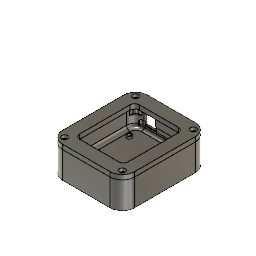
box (Autodesk Fusion 360 design; units mm, degrees)
Autodesk Fusion 360 part; units mm, degrees
sketch "Sketch1" plane through (0, 0, 2.8) normal (0, 0, 1) x (-1, 0, 0)
  circle A0 centre (-2.5, -2.5) radius 1.15 construction
  circle A1 centre (-48.5, -2.5) radius 1.15 construction
  circle A2 centre (-48.5, -61.5) radius 1.15 construction
  circle A3 centre (-2.5, -61.5) radius 1.15 construction
  line L0 (-2.5, -73.5) -> (-48.5, -73.5)
  line L1 (-60.5, -61.5) -> (-60.5, -2.5)
  line L2 (-48.5, 9.5) -> (-2.5, 9.5)
  line L3 (9.5, -2.5) -> (9.5, -61.5)
  arc A4 (-2.5, -73.5) -> (9.5, -61.5) centre (-2.5, -61.5) ccw
  arc A5 (-60.5, -61.5) -> (-48.5, -73.5) centre (-48.5, -61.5) ccw
  arc A6 (-48.5, 9.5) -> (-60.5, -2.5) centre (-48.5, -2.5) ccw
  arc A7 (9.5, -2.5) -> (-2.5, 9.5) centre (-2.5, -2.5) ccw
  arc A8 (-2.5, -7.5) -> (-6.5, -3.5) centre (-6.5, -7.5) ccw
  line L4 (-6.5, -3.5) -> (-44.5, -3.5)
  arc A9 (-44.5, -3.5) -> (-48.5, -7.5) centre (-44.5, -7.5) ccw
  line L5 (-48.5, -7.5) -> (-48.5, -56.5)
  arc A10 (-48.5, -56.5) -> (-44.5, -60.5) centre (-44.5, -56.5) ccw
  line L6 (-44.5, -60.5) -> (-6.5, -60.5)
  arc A11 (-6.5, -60.5) -> (-2.5, -56.5) centre (-6.5, -56.5) ccw
  line L7 (-2.5, -56.5) -> (-2.5, -7.5)
  line L8 (-44.5, -61) -> (-6.5, -61)
  arc A12 (-6.5, -61) -> (-2, -56.5) centre (-6.5, -56.5) ccw
  line L9 (-2, -56.5) -> (-2, -7.5)
  arc A13 (-2, -7.5) -> (-6.5, -3) centre (-6.5, -7.5) ccw
  line L10 (-6.5, -3) -> (-44.5, -3)
  arc A14 (-44.5, -3) -> (-49, -7.5) centre (-44.5, -7.5) ccw
  line L11 (-49, -7.5) -> (-49, -56.5)
  arc A15 (-49, -56.5) -> (-44.5, -61) centre (-44.5, -56.5) ccw
  circle A16 centre (-2.5, -61.5) radius 1.25
  circle A17 centre (-48.5, -61.5) radius 1.25
  circle A18 centre (-48.5, -2.5) radius 1.25
  circle A19 centre (-2.5, -2.5) radius 1.25
  dimension "d1" = 12
  dimension "d3" = 0.5
  dimension "d6" = 2.5
  dimension "d7" = 2.5
  dimension "d8" = 2.5
  dimension "d9" = 2.5
  measures "d1" radius of A4
  measures "d6" diameter of A16
  measures "d7" diameter of A17
  measures "d8" diameter of A19
  measures "d9" diameter of A18
extrude "Extrude1" add sketch "Sketch1" along normal blind 4.5 contours L0 L1 L2 L3 A4 A5 A6 A7 | A16 | A17 | A18 | A19 makes body 1
extrude "Extrude2" cut sketch "Sketch1" along normal blind 3.4 contours A16 | A17 | A18 | A19 bodies 1
ref_plane "WorkPlane1" through (25.5, 32, -23.2) normal (0, 0, -1) x (1, 0, 0)
sketch "Sketch2" plane through (25.5, 32, -23.2) normal (0, 0, -1) x (1, 0, 0)
  arc A0 (-35, -29.5) -> (-23, -41.5) centre (-23, -29.5) ccw
  line L0 (-23, -41.5) -> (23, -41.5)
  arc A1 (23, -41.5) -> (35, -29.5) centre (23, -29.5) ccw
  line L1 (35, -29.5) -> (35, 29.5)
  arc A2 (35, 29.5) -> (23, 41.5) centre (23, 29.5) ccw
  line L2 (23, 41.5) -> (-23, 41.5)
  arc A3 (-23, 41.5) -> (-35, 29.5) centre (-23, 29.5) ccw
  line L3 (-35, 29.5) -> (-35, -29.5)
extrude "Extrude3" add sketch "Sketch2" against normal up to surface (26 mm away) separate body makes body 2
shell "Shell1" thickness 3 removed faces 1 at (37.1667, 22.1667, 2.8) on bodies 2
fillet "Fillet1" radius 3.5 8 edges at (-3.864, -3.864, -20.2) (-6.5, 32, -20.2) (-3.864, 67.864, -20.2) (25.5, 70.5, -20.2) (54.864, 67.864, -20.2) (57.5, 32, -20.2) (54.864, -3.864, -20.2) (25.5, -6.5, -20.2) on bodies 2
ref_plane "WorkPlane2" through (25.5, 32, -18.2) normal (0, 0, 1) x (-1, 0, 0)
ref_plane "WorkPlane3" through (25.5, 32, -10.2) normal (1, 0, 0) x (0, 1, 0)
sketch "Sketch3" plane through (25.5, 32, -18.2) normal (0, 0, 1) x (1, 0, 0)
  line L0 (26.65, -26.3) -> (26.65, 38)
  arc A0 (26.65, 38) -> (26.15, 38.5) centre (26.15, 38) ccw
  line L1 (26.15, 38.5) -> (13.95, 38.5)
  line L2 (9.35, 38.5) -> (-13.85, 38.5)
  line L3 (-22.85, 38.5) -> (-26.15, 38.5)
  line L4 (-26.65, 38) -> (-26.65, -27)
  arc A1 (-26.15, 38.5) -> (-26.65, 38) centre (-26.15, 38) ccw
  line L5 (-22.85, 38.5) -> (-13.85, 38.5)
  line L6 (9.35, 38.5) -> (13.95, 38.5)
  line L7 (27.85, -26.3) -> (27.85, 38)
  arc A2 (27.85, 38) -> (26.15, 39.7) centre (26.15, 38) ccw
  line L8 (26.15, 39.7) -> (13.95, 39.7)
  line L9 (9.35, 39.7) -> (13.95, 39.7)
  line L10 (9.35, 39.7) -> (-13.85, 39.7)
  line L11 (-22.85, 39.7) -> (-13.85, 39.7)
  line L12 (-22.85, 39.7) -> (-26.15, 39.7)
  arc A3 (-26.15, 39.7) -> (-27.85, 38) centre (-26.15, 38) ccw
  line L13 (-27.85, 38) -> (-27.85, -27)
  line L14 (26.65, -26.3) -> (27.85, -26.3)
  line L15 (-27.85, -27) -> (-26.65, -27)
  line L16 (26.65, -26.3) -> (-26.65, -27)
  dimension "d26" = 1.2
extrude "Extrude4" cut sketch "Sketch3" along normal blind 5 bodies 2
sketch "Sketch4" plane through (0, 73.5, 0) normal (0, 1, 0) x (-1, 0, 0)
  line L0 (-2.65, -16.4) -> (-2.65, -4.9) construction
  line L1 (-2.65, -4.9) -> (-11.65, -4.9) construction
  line L2 (-11.65, -4.9) -> (-11.65, -16.4) construction
  line L3 (-11.65, -16.4) -> (-2.65, -16.4) construction
  line L4 (-40.85, -14.9) -> (-40.85, -14.4)
  line L5 (-33.35, -14.9) -> (-33.35, -14.4)
  line L6 (-39.45, -13.4) -> (-34.85, -13.4)
  line L7 (-34.85, -16.4) -> (-39.45, -16.4)
  line L8 (-1.65, -17.4) -> (-1.65, -3.9)
  line L9 (-1.65, -3.9) -> (-12.65, -3.9)
  line L10 (-12.65, -3.9) -> (-12.65, -17.4)
  line L11 (-12.65, -17.4) -> (-1.65, -17.4)
  line L12 (-42.35, -17.9) -> (-42.35, -11.9)
  line L13 (-42.35, -11.9) -> (-31.85, -11.9)
  line L14 (-31.85, -11.9) -> (-31.85, -17.9)
  line L15 (-42.35, -17.9) -> (-31.85, -17.9)
  dimension "d29" = 1
  dimension "d31" = 1.5
  dimension "d32" = 1.5
  dimension "d33" = 1.5
  dimension "d34" = 1.5
  measures "d31" distance of L7 L15
  measures "d32" distance of L6 L13
  measures "d33" distance of L5 L14
  measures "d34" distance of L4 L12
extrude "Extrude5" cut sketch "Sketch4" against normal up to surface (5 mm away) bodies 2
sketch "Sketch5" plane through (0, 0, -20.2) normal (0, 0, 1) x (-1, 0, 0)
  circle A0 centre (-6.65, -4.3) radius 1.5
  circle A1 centre (-1.35, -56.5) radius 1.5
  circle A2 centre (-49.65, -55.5) radius 1.5
  circle A3 centre (-34.65, -4.3) radius 1.5
  circle A4 centre (-34.65, -4.3) radius 2.5
  circle A5 centre (-6.65, -4.3) radius 2.5
  circle A6 centre (-1.35, -56.5) radius 2.5
  circle A7 centre (-49.65, -55.5) radius 2.5
  dimension "d37" = 1
  dimension "d38" = 1
  dimension "d39" = 1
  dimension "d40" = 1
extrude "Extrude6" add sketch "Sketch5" along normal up to surface (2 mm away) bodies 2
extrude "Extrude7" cut sketch "Sketch5" against normal up to surface (3 mm away) contours A0 | A1 | A2 | A3 bodies 2
sketch "Sketch6" plane through (0, 0, 7.3) normal (0, 0, 1) x (-1, 0, 0)
  circle A0 centre (2.5, 2.5) radius 2.9
  circle A1 centre (-53.5, 2.5) radius 2.9
  circle A2 centre (-53.5, -66.5) radius 2.9
  circle A3 centre (2.5, -66.5) radius 2.9
  line L0 (-2.5, 9.5) -> (-48.5, 9.5)
  line L1 (9.5, -61.5) -> (9.5, -2.5)
  line L2 (-60.5, -2.5) -> (-60.5, -61.5)
  line L3 (-48.5, -73.5) -> (-2.5, -73.5)
  circle A4 centre (-53.5, 2.5) radius 1.7
  circle A5 centre (2.5, 2.5) radius 1.7
  circle A6 centre (2.5, -66.5) radius 1.7
  circle A7 centre (-53.5, -66.5) radius 1.7
  dimension "d45" = 5.8
  dimension "d46" = 5.8
  dimension "d47" = 5.8
  dimension "d48" = 5.8
  dimension "d49" = 7
  dimension "d50" = 7
  dimension "d51" = 7
  dimension "d52" = 7
  dimension "d55" = 3.4
  dimension "d56" = 3.4
  dimension "d57" = 3.4
  dimension "d58" = 3.4
  measures "d45" diameter of A0
  measures "d46" diameter of A1
  measures "d47" diameter of A2
  measures "d48" diameter of A3
  measures "d49" distance of A0.centre L0
  measures "d50" distance of A0.centre L1
  measures "d51" distance of A1.centre L2
  measures "d52" distance of A3.centre L3
  measures "d55" diameter of A4
  measures "d56" diameter of A5
  measures "d57" diameter of A7
  measures "d58" diameter of A6
extrude "Extrude8" cut sketch "Sketch6" against normal blind 3 contours A0 | A1 | A2 | A3 | A4 | A5 | A6 | A7 bodies 1
extrude "Extrude9" cut sketch "Sketch6" against normal up to surface (4.5 mm away) contours A4 | A5 | A6 | A7 bodies 1
ref_plane "WorkPlane4" through (25.5, 32, -10.2) normal (0, -1, 0) x (1, 0, 0)
sketch "Sketch7" plane through (0, 0, 2.8) normal (0, 0, -1) x (1, 0, 0)
  circle A0 centre (-2.5, 2.5) radius 1.7
  circle A1 centre (-2.5, -66.5) radius 1.7
  circle A2 centre (53.5, -66.5) radius 1.7
  circle A3 centre (53.5, 2.5) radius 1.7
  circle A4 centre (53.5, -66.5) radius 1.5
  circle A5 centre (53.5, 2.5) radius 1.5
  circle A6 centre (-2.5, 2.5) radius 1.5
  circle A7 centre (-2.5, -66.5) radius 1.5
  circle A8 centre (53.5, 2.5) radius 2.5
  arc A9 (57.5, -2.5) -> (48.5, 6.5) centre (48.5, -2.5) ccw
  line L0 (53.5, 0) -> (57.1458, 0)
  line L1 (51, 2.5) -> (51, 6.1458)
  line L2 (25.5, 3.4) -> (25.5, -80.4837)
  line L3 (-2.5, 0) -> (-6.1458, 0)
  circle A10 centre (-2.5, 2.5) radius 2.5
  line L4 (0, 2.5) -> (0, 6.1458)
  line L5 (-2.1, -32) -> (53.1, -32)
  line L6 (53.5, -64) -> (57.1458, -64)
  circle A11 centre (53.5, -66.5) radius 2.5
  line L7 (51, -66.5) -> (51, -70.1458)
  line L8 (0, -66.5) -> (0, -70.1458)
  circle A12 centre (-2.5, -66.5) radius 2.5
  line L9 (-2.5, -64) -> (-6.1458, -64)
  arc A13 (2.5, 6.5) -> (-6.5, -2.5) centre (2.5, -2.5) ccw
  arc A14 (-6.5, -61.5) -> (2.5, -70.5) centre (2.5, -61.5) ccw
  arc A15 (48.5, -70.5) -> (57.5, -61.5) centre (48.5, -61.5) ccw
  dimension "d61" = 3
  dimension "d62" = 3
  dimension "d63" = 3
  dimension "d64" = 3
  dimension "d65" = 1
  measures "d61" diameter of A4
  measures "d62" diameter of A7
  measures "d63" diameter of A5
  measures "d64" diameter of A6
  measures "d65" distance of A5 A8
extrude "Extrude10" add sketch "Sketch7" along normal blind 8 separate body contours A0 | A1 | A2 | A3 | A4 | A5 | A6 | A7 | A8 A9 | A8 A9 L1 | A8 A9 L0 | A10 A13 | L3 A10 A13 | A10 L4 A13 | A11 A15 | L6 A11 A15 | A11 L7 A15 | A12 A14 | L8 A12 A14 | A12 L9 A14 picked at (53.9267, 4.4768) picked at (-2.9267, 4.4768) picked at (53.9267, -68.4768) picked at (-2.9267, -68.4768) makes body 3 at (54.7094, -4.0148, -2.5333) makes body 4 at (-4.5799, -3.0565, 0.1333) makes body 5 at (54.7094, 68.0148, 0.1333) makes body 6 at (-1.6036, 69.51, -2.5333)
combine "Combine2" operation add target body 2 tool bodies 4 3 5 6
chamfer "Chamfer1" distance 4.4 angle 45 4 edges at (-3.864, 67.864, -5.2) (-3.864, -3.864, -5.2) (54.864, -3.864, -5.2) (54.864, 67.864, -5.2) on bodies 2
extrude "Extrude11" cut sketch "Sketch7" along normal blind 9 contours A4 | A5 | A6 | A7 bodies 2
chamfer "Chamfer2" distance 1.2 angle 45 7 edges at (0.5, 71.7, -13.2) (-1.8521, 71.2021, -13.2) (-2.35, 69.5407, -13.2) (22.25, 71.7, -13.2) (53.35, 69.5407, -13.2) (52.8521, 71.2021, -13.2) (47, 71.7, -13.2) on bodies 2
equation "d7 = d6"
equation "d8 = d6"
equation "d9 = d6"
equation "d12 = 22 mm + 4 mm"
equation "d32 = d31"
equation "d34 = d33"
equation "d38 = d37"
equation "d39 = d37"
equation "d40 = d37"
equation "d46 = d45"
equation "d47 = d45"
equation "d48 = d45"
equation "d50 = d49"
equation "d51 = d49"
equation "d52 = d49"
equation "d56 = d55"
equation "d57 = d55"
equation "d58 = d55"
equation "d62 = d61"
equation "d63 = d61"
equation "d64 = d61"
